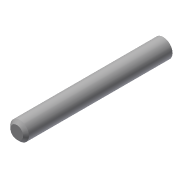
# Autodesk Inventor part: 1.FRP.000.006.ipt
Saved by Autodesk Inventor 2021 (Build 250183000, 183)
## iProperties
Created: 2023-12-12
Part Number: 1.FRP.000.006.ipt
Material: ASTM A36
Document SubType Name: Modeling
Designer: RICARDO MOREIRA
Density: 7.85 g/cm^3
Appearance: Steel
Description: BARRA FAB REDONDA ASTM A36 12,7X12,7X100
Mass: 98.8807 g
Surface Area: 41.9123 cm^2
Volume: 12.5963 cm^3
0_GRUPO: 0_BARRA FAB
1_MODIFICADOR: 1_REDONDA
2_MATERIAL: ASTM A36
4_MEDIDA X: 12,7
5_MEDIDA Y: 12,7
6_MEDIDA Z: 100
Author: RICARDO MOREIRA
Autodesk Inventor part; units mm, degrees
sketch "Sketch1" plane through (0, 0, 0) normal (0, 0, 1) x (1, 0, 0)
  circle A0 centre (0, 0) radius 6.35
  dimension "d1" = 12.7
  constraints: 1 centre point, 1 coincident
  measures "d1" diameter of A0
extrude "Extrusion1" add sketch "Sketch1" along normal mid plane 100
chamfer "Chamfer1" distance 2 angle 45 1 edges at (-6.35, 0, 50)
body "Solid1"
